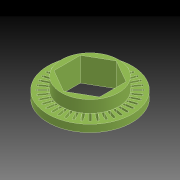
# Autodesk Inventor part: KB33-046-002-004 - Колесо энкодера
Saved by Autodesk Inventor 2020 (Build 240168000, 168)
## iProperties
Created: 2021-07-26
Part Number: KB33-046-002-004 - Колесо энкодера
Material: Типовые
Document SubType Name: Modeling
Designer: Петров Иван
Mass: 2.40692 g
Surface Area: 36.2467 cm^2
Volume: 2.40692 cm^3
Density: 1 g/cm^3
Appearance: Оливково-зеленый
Author: Петров Иван
Autodesk Inventor part; units mm, degrees
ref_plane "YZ Plane" through (0, 0, 0) normal (1, 0, 0) x (0, 1, 0)
ref_plane "XZ Plane" through (0, 0, 0) normal (0, 1, 0) x (-1, 0, 0)
ref_plane "XY Plane" through (0, 0, 0) normal (0, 0, 1) x (1, 0, 0)
sketch "Эскиз1" plane through (0, 0, 0) normal (0, 1, 0) x (-1, 0, 0)
  circle A0 centre (0, 0) radius 6
  circle A1 centre (0, 0) radius 17.5
  dimension "d0" = 12
  dimension "d1" = 35
  constraints: 2 centre point, 2 coincident
  measures "d0" diameter of A0
  measures "d1" diameter of A1
extrude "Выдавливание1" add sketch "Эскиз1" along normal blind 3
sketch "Эскиз2" plane through (0, 3, 0) normal (0, 1, 0) x (1, 0, 0)
  line L0 (-12.4371, 0) -> (-15.5629, 0) construction
  line L1 (-12.4371, 0.5) -> (-15.5629, 0.5)
  line L2 (-15.5629, -0.5) -> (-12.4371, -0.5)
  arc A0 (-12.4371, -0.5) -> (-12.4371, 0.5) centre (-12.4371, 0) ccw
  arc A1 (-15.5629, 0.5) -> (-15.5629, -0.5) centre (-15.5629, 0) ccw
  point P0 (0, 0)
  point P1 (-14, 0)
  dimension "d4" = 1
  dimension "d10" = 14
  constraints: 8 end point, 4 point on circle, 4 tangent, 2 centre point, 1 horizontal, 1 midpoint, 1 parallel
  measures "d4" diameter of A1
  measures "d10" distance of point (0, 0) point (-14, 0)
extrude "Выдавливание2" cut sketch "Эскиз2" against normal blind 3
pattern_circular "Круговой массив1" count 40 over 360 about axis through (0, 0, 0) along (0, 1, 0) of "Выдавливание2"
sketch "Эскиз3" plane through (0, 3, 0) normal (0, 1, 0) x (1, 0, 0)
  line L0 (0, 11) -> (9.5263, 5.5)
  line L1 (9.5263, 5.5) -> (9.5263, -5.5)
  line L2 (9.5263, -5.5) -> (0, -11)
  line L3 (0, -11) -> (-9.5263, -5.5)
  line L4 (-9.5263, -5.5) -> (-9.5263, 5.5)
  line L5 (-9.5263, 5.5) -> (0, 11)
  circle A0 centre (0, 0) radius 11.9371
  arc A1 (-0.5, 12.4371) -> (0.5, 12.4371) centre (0, 12.4371) ccw projected
  point P0 (0, 0)
  point P1 (0, 0)
  dimension "d11" = 22
  constraints: 12 end point, 1 centre point, 1 coincident, 1 tangent, 13 other
  measures "d11" distance of L2.end L0.start
extrude "Выдавливание3" add sketch "Эскиз3" along normal mid plane 10
sketch "Эскиз4" plane through (0, 3, 0) normal (0, 1, 0) x (1, 0, 0)
  line L0 (-9.5263, 5.5) -> (-9.5263, -5.5) projected
  line L1 (-9.5263, -5.5) -> (0, -11) projected
  line L2 (0, -11) -> (9.5263, -5.5) projected
  line L3 (9.5263, -5.5) -> (9.5263, 5.5) projected
  line L4 (9.5263, 5.5) -> (0, 11) projected
  line L5 (0, 11) -> (-9.5263, 5.5) projected
  circle A0 centre (0, 0) radius 6 projected
extrude "Выдавливание4" cut sketch "Эскиз4" against normal blind 10
